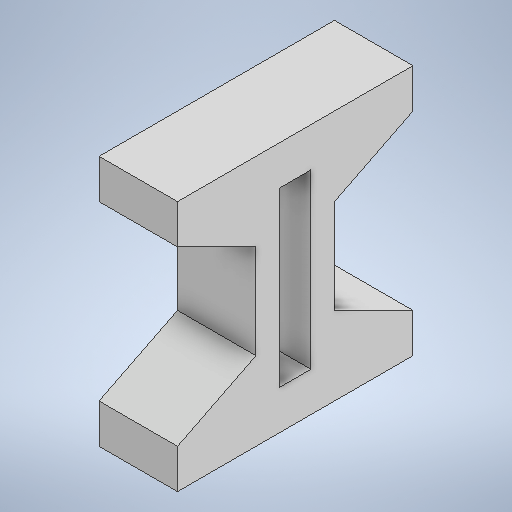
# Autodesk Inventor part: stand
Saved by Autodesk Inventor 2025.2 (Build 292293000, 293)
## iProperties
Created: 2025-04-10
Part Number: stand
Material: Generic
Document SubType Name: Modeling
Designer: joaki
Density: 1 g/cm^3
Appearance: Default
Author: joaki
Autodesk Inventor part; units mm, degrees
ref_plane "YZ Plane" through (0, 0, 0) normal (1, 0, 0) x (0, 1, 0)
ref_plane "XZ Plane" through (0, 0, 0) normal (0, 1, 0) x (-1, 0, 0)
ref_plane "XY Plane" through (0, 0, 0) normal (0, 0, 1) x (1, 0, 0)
sketch "Sketch1" plane through (0, 0, 0) normal (0, 1, 0) x (-1, 0, 0)
  line L0 (4.2334, 3.223) -> (-5.7666, 3.223)
  line L1 (-5.7666, 3.223) -> (-5.7666, -6.777)
  line L2 (-5.7666, -6.777) -> (4.2334, -6.777)
  line L3 (4.2334, -6.777) -> (4.2334, 3.223)
  point P0 (0, 0)
  dimension "d0" = 10
  dimension "d1" = 10
  constraints: 8 end point, 2 parallel, 1 horizontal, 1 perpendicular
  measures "d0" distance between parallel lines of L1 L3
  measures "d1" distance of L2.end L0.start
extrude "Extrusion1" add sketch "Sketch1" along normal blind 32
sketch "Sketch2" plane through (5.7666, 0, 3.223) normal (1, 0, 0) x (0, 0, -1)
  line L0 (0, 0) -> (10, 0) projected
  line L1 (0, 0) -> (0, 32) projected
  line L2 (10, 0) -> (0, 0)
  line L3 (0, 0) -> (0, 10)
  line L4 (0, 10) -> (10, 10)
  line L5 (10, 10) -> (10, 0)
  line L6 (0, 0) -> (-10, 0)
  line L7 (-10, 0) -> (-10, 10)
  line L8 (-10, 10) -> (0, 10)
  line L9 (0, 10) -> (0, 0)
  line L10 (10, 10) -> (20, 10)
  line L11 (20, 10) -> (20, 0)
  line L12 (20, 0) -> (10, 0)
  line L13 (10, 0) -> (10, 10)
  line L14 (-10, 5) -> (0, 10)
  line L15 (10, 10) -> (20, 5)
  point P0 (3.223, 0)
  point P1 (10, 5)
  dimension "d4" = 10
  dimension "d5" = 10
  dimension "d6" = 10
  constraints: 28 end point, 6 parallel, 3 horizontal, 3 midpoint, 3 perpendicular, 2 point on line
  measures "d4" distance between parallel lines of L0 L4
  measures "d5" distance from line of L1 L14.start
  measures "d6" distance of point (10, 5) L15.end
extrude "Extrusion2" add sketch "Sketch2" against normal blind 10 contours L6 L7 L14 L1 | L5 L15 L11 L12
sketch "Sketch3" plane through (5.7666, 32, 3.223) normal (1, 0, 0) x (0, 0, -1)
  line L0 (10, 0) -> (0, 0) projected
  line L1 (10, -22) -> (10, 0) projected
  line L2 (0, 0) -> (10, 0)
  line L3 (10, 0) -> (10, -10)
  line L4 (10, -10) -> (0, -10)
  line L5 (0, -10) -> (0, 0)
  line L6 (0, 0) -> (-10, 0)
  line L7 (-10, 0) -> (-10, -10)
  line L8 (-10, -10) -> (0, -10)
  line L9 (0, -10) -> (0, 0)
  line L10 (10, 0) -> (20, 0)
  line L11 (20, 0) -> (20, -10)
  line L12 (20, -10) -> (10, -10)
  line L13 (10, -10) -> (10, 0)
  line L14 (0, -10) -> (-10, -5)
  line L15 (10, -10) -> (20, -5)
  point P0 (3.223, -32)
  point P1 (0, -10)
  dimension "d9" = 10
  dimension "d10" = 10
  dimension "d11" = 10
  constraints: 28 end point, 6 parallel, 3 horizontal, 3 perpendicular, 2 midpoint, 2 point on line
  measures "d9" distance between parallel lines of L0 L4
  measures "d10" distance between parallel lines of L1 L11
  measures "d11" distance between parallel lines of L5 L7
extrude "Extrusion3" add sketch "Sketch3" against normal blind 10 contours L10 L11 L15 L1 | L5 L14 L7 L6
sketch "Sketch4" plane through (5.7666, 0, -16.777) normal (1, 0, 0) x (0, 0, -1)
  line L0 (-13, 27) -> (-17, 27)
  line L1 (-17, 27) -> (-17, 5)
  line L2 (-17, 5) -> (-13, 5)
  line L3 (-13, 5) -> (-13, 27)
  line L4 (0, 32) -> (-30, 32) projected
  line L5 (-30, 0) -> (0, 0) projected
  line L6 (-10, 10) -> (-10, 22) projected
  line L7 (-20, 10) -> (-20, 22) projected
  point P0 (-16.777, 0)
  point P1 (-15, 32)
  point P2 (-15, 27)
  point P3 (-15, 5)
  dimension "d14" = 5
  dimension "d15" = 5
  dimension "d16" = 3
  dimension "d17" = 3
  constraints: 8 end point, 3 midpoint, 2 parallel, 1 horizontal, 1 perpendicular
  measures "d14" distance of point (-15, 32) point (-15, 27)
  measures "d15" distance from line of L5 point (-15, 5)
  measures "d16" distance between parallel lines of L6 L3
  measures "d17" distance between parallel lines of L7 L1
extrude "Extrusion4" cut sketch "Sketch4" against normal blind 10
body "Solid1"
